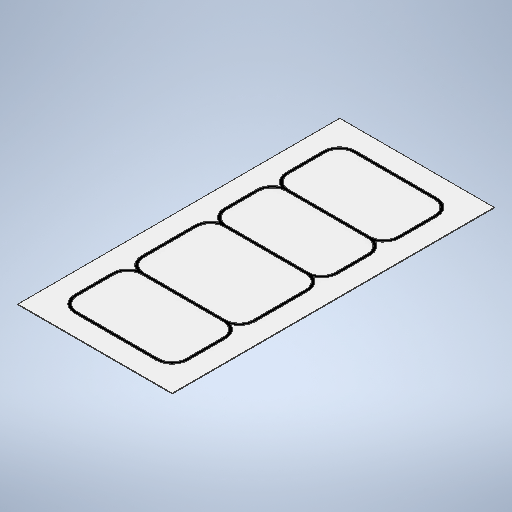
# Autodesk Inventor part: pista
Saved by Autodesk Inventor 2025.2 (Build 292293000, 293)
## iProperties
Created: 2025-11-10
Part Number: pista
Material: Genérico
Document SubType Name: Modeling
Designer: Dax
Density: 1 g/cm^3
Appearance: Valor por defecto
Author: Dax
Autodesk Inventor part; units mm, degrees
ref_plane "YZ Plane" through (0, 0, 0) normal (1, 0, 0) x (0, 1, 0)
ref_plane "XZ Plane" through (0, 0, 0) normal (0, 1, 0) x (-1, 0, 0)
ref_plane "XY Plane" through (0, 0, 0) normal (0, 0, 1) x (1, 0, 0)
sketch "Boceto1" plane through (0, 0, 0) normal (0, 1, 0) x (-1, 0, 0)
  line L0 (120, 0) -> (708.2202, 0)
  line L1 (0, -120) -> (0, -516)
  line L2 (120, -616) -> (390.8035, -616)
  line L3 (0, -736) -> (0, -978)
  line L4 (120, -1078) -> (730, -1078)
  line L5 (850, -736) -> (850, -978)
  line L6 (850, -516) -> (850, -120)
  line L7 (0, -1198) -> (0, -1498)
  line L8 (120, -1578) -> (730, -1578)
  line L9 (850, -1478) -> (850, -1198)
  line L10 (0, 100) -> (0, 380)
  line L11 (120, 500) -> (730, 500)
  line L12 (730, 0) -> (708.2202, 0)
  line L13 (850, 380) -> (850, 100)
  line L14 (830, 100) -> (830, 380)
  line L15 (730, 480) -> (120, 480)
  line L16 (20, 380) -> (20, 100)
  line L17 (120, -20) -> (708.2202, -20)
  line L18 (708.2202, -20) -> (730, -20)
  line L19 (120, -636) -> (730, -636)
  line L20 (120, -1098) -> (730, -1098)
  line L21 (750, -1598) -> (100, -1598)
  line L22 (20, -120) -> (20, -516)
  line L23 (20, -736) -> (20, -978)
  line L24 (20, -1198) -> (20, -1478)
  line L25 (830, -1478) -> (830, -1198)
  line L26 (830, -736) -> (830, -978)
  line L27 (830, -516) -> (830, -120)
  arc A0 (20, -1478) -> (120, -1578) centre (120, -1478) ccw
  arc A1 (730, -1578) -> (830, -1478) centre (730, -1478) ccw
  arc A2 (830, -1198) -> (730, -1098) centre (730, -1198) ccw
  arc A3 (730, -1078) -> (830, -978) centre (730, -978) ccw
  arc A4 (830, -736) -> (730, -636) centre (730, -736) ccw
  arc A5 (730, -616) -> (830, -516) centre (730, -516) ccw
  arc A6 (830, -120) -> (730, -20) centre (730, -120) ccw
  arc A7 (730, 0) -> (830, 100) centre (730, 100) ccw
  arc A8 (830, 380) -> (730, 480) centre (730, 380) ccw
  arc A9 (120, 480) -> (20, 380) centre (120, 380) ccw
  arc A10 (20, 100) -> (120, 0) centre (120, 100) ccw
  arc A11 (120, -20) -> (20, -120) centre (120, -120) ccw
  arc A12 (20, -516) -> (120, -616) centre (120, -516) ccw
  arc A13 (120, -636) -> (20, -736) centre (120, -736) ccw
  arc A14 (20, -978) -> (120, -1078) centre (120, -978) ccw
  arc A15 (120, -1098) -> (20, -1198) centre (120, -1198) ccw
  line L28 (850, -978) -> (850, -736)
  arc A16 (850, -736) -> (777.9583, -626) centre (730, -736) ccw
  line L29 (730, -616) -> (120, -616)
  arc A17 (72.0417, -626) -> (0, -736) centre (120, -736) ccw
  line L30 (0, -736) -> (0, -978)
  arc A18 (0, -978) -> (72.0417, -1088) centre (120, -978) ccw
  line L31 (120, -1098) -> (730, -1098)
  arc A19 (777.9583, -1088) -> (850, -978) centre (730, -978) ccw
  line L32 (850, -1198) -> (850, -1478)
  arc A20 (730, -1598) -> (850, -1478) centre (730, -1478) ccw
  line L33 (730, -1598) -> (120, -1598)
  arc A21 (0, -1478) -> (120, -1598) centre (120, -1478) ccw
  line L34 (0, -1478) -> (0, -1198)
  arc A22 (72.0417, -1088) -> (0, -1198) centre (120, -1198) ccw
  line L35 (120, -1078) -> (730, -1078)
  arc A23 (850, -1198) -> (777.9583, -1088) centre (730, -1198) ccw
  line L36 (390.8035, -636) -> (120, -636)
  arc A24 (0, -516) -> (72.0417, -626) centre (120, -516) ccw
  line L37 (0, -516) -> (0, -120)
  arc A25 (72.0417, -10) -> (0, -120) centre (120, -120) ccw
  line L38 (120, 0) -> (708.2202, 0)
  line L39 (708.2202, 0) -> (730, 0)
  arc A26 (850, -120) -> (777.9583, -10) centre (730, -120) ccw
  line L40 (850, -120) -> (850, -516)
  arc A27 (777.9583, -626) -> (850, -516) centre (730, -516) ccw
  line L41 (850, 380) -> (850, 100)
  arc A28 (777.9583, -10) -> (850, 100) centre (730, 100) ccw
  line L42 (730, -20) -> (708.2202, -20)
  line L43 (708.2202, -20) -> (120, -20)
  arc A29 (0, 100) -> (72.0417, -10) centre (120, 100) ccw
  line L44 (0, 100) -> (0, 380)
  arc A30 (120, 500) -> (0, 380) centre (120, 380) ccw
  line L45 (120, 500) -> (730, 500)
  arc A31 (850, 380) -> (730, 500) centre (730, 380) ccw
  point P0 (0, 500)
  point P1 (0, -1478)
  point P2 (730, -1598)
  constraints: 92 end point, 64 point on circle, 32 centre point, 31 tangent, 15 equal radius, 6 perpendicular, 5 parallel, 4 vertical, 2 point on line, 1 collinear, 1 horizontal, 9 other
extrude "Extrusión1" add sketch "Boceto1" along normal blind 6
sketch "Boceto2" plane through (0, 0, 0) normal (0, -1, 0) x (1, 0, 0)
  line L0 (-1000, 500) -> (-1000, -1750)
  line L1 (-1000, -1750) -> (0, -1750)
  line L2 (152, 652) -> (-1000, 652)
  line L3 (152, -1750) -> (152, 652)
  line L4 (-1000, 500) -> (-1000, 652)
  line L5 (0, -1750) -> (152, -1750)
  point P0 (0, 0)
  constraints: 12 end point, 2 perpendicular
extrude "Extrusión2" add sketch "Boceto2" against normal blind 5
